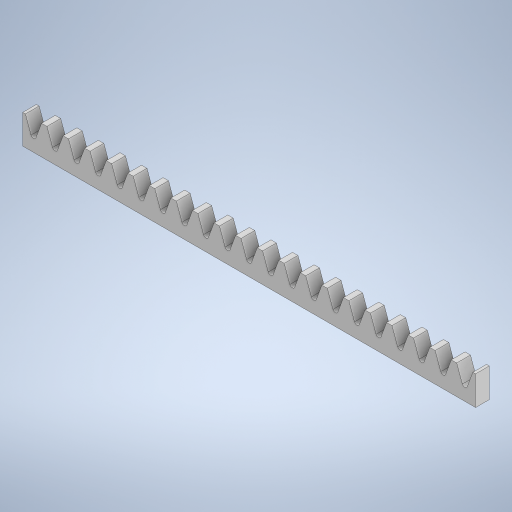
# Autodesk Inventor part: 齒條
Saved by Autodesk Inventor 2024 (Build 280153000, 153)
## iProperties
Created: 2024-04-20
Part Number: 齒條
Material: 一般
Document SubType Name: Modeling
Designer: rumse
Density: 1 g/cm^3
Appearance: 預設
Author: rumse
Autodesk Inventor part; units mm, degrees
note: some values were not read from the file. Left out: dimensions or parameters whose unit could not be read.
ref_plane "YZ Plane" through (0, 0, 0) normal (1, 0, 0) x (0, 1, 0)
ref_plane "XZ Plane" through (0, 0, 0) normal (0, 1, 0) x (-1, 0, 0)
ref_plane "XY Plane" through (0, 0, 0) normal (0, 0, 1) x (1, 0, 0)
sketch "草圖2" plane through (0, 0, 0) normal (0, 0, 1) x (1, 0, 0)
  line L0 (0, 0) -> (32.9867, 0)
  line L1 (32.9867, 0) -> (32.9867, 2.125)
  line L2 (32.9867, 2.125) -> (0, 2.125)
  line L3 (0, 2.125) -> (0, 0)
  line L4 (0, 1) -> (32.9867, 1) construction
  line L5 (0.1974, 2.125) -> (0.6069, 1)
  line L6 (0.9639, 1) -> (1.3734, 2.125)
  line L7 (0.7854, 2.125) -> (0.7854, 1) construction
  line L8 (0, 0.875) -> (32.9867, 0.875) construction
  arc A0 (0.6069, 1) -> (0.9639, 1) centre (0.7854, 1.065) ccw
  line L9 (0, 1.625) -> (32.9867, 1.625) construction
  line L10 (2.5347, 1) -> (2.9442, 2.125)
  arc A1 (2.1777, 1) -> (2.5347, 1) centre (2.3562, 1.065) ccw
  line L11 (1.7682, 2.125) -> (2.1777, 1)
  line L12 (4.1055, 1) -> (4.515, 2.125)
  arc A2 (3.7484, 1) -> (4.1055, 1) centre (3.927, 1.065) ccw
  line L13 (3.339, 2.125) -> (3.7484, 1)
  line L14 (5.6763, 1) -> (6.0858, 2.125)
  arc A3 (5.3192, 1) -> (5.6763, 1) centre (5.4978, 1.065) ccw
  line L15 (4.9098, 2.125) -> (5.3192, 1)
  line L16 (7.2471, 1) -> (7.6566, 2.125)
  arc A4 (6.89, 1) -> (7.2471, 1) centre (7.0686, 1.065) ccw
  line L17 (6.4806, 2.125) -> (6.89, 1)
  line L18 (8.8179, 1) -> (9.2274, 2.125)
  arc A5 (8.4608, 1) -> (8.8179, 1) centre (8.6394, 1.065) ccw
  line L19 (8.0514, 2.125) -> (8.4608, 1)
  line L20 (10.3887, 1) -> (10.7982, 2.125)
  arc A6 (10.0316, 1) -> (10.3887, 1) centre (10.2102, 1.065) ccw
  line L21 (9.6222, 2.125) -> (10.0316, 1)
  line L22 (11.9595, 1) -> (12.369, 2.125)
  arc A7 (11.6024, 1) -> (11.9595, 1) centre (11.781, 1.065) ccw
  line L23 (11.193, 2.125) -> (11.6024, 1)
  line L24 (13.5303, 1) -> (13.9398, 2.125)
  arc A8 (13.1732, 1) -> (13.5303, 1) centre (13.3518, 1.065) ccw
  line L25 (12.7638, 2.125) -> (13.1732, 1)
  line L26 (15.1011, 1) -> (15.5106, 2.125)
  arc A9 (14.744, 1) -> (15.1011, 1) centre (14.9226, 1.065) ccw
  line L27 (14.3346, 2.125) -> (14.744, 1)
  line L28 (16.6719, 1) -> (17.0814, 2.125)
  arc A10 (16.3148, 1) -> (16.6719, 1) centre (16.4934, 1.065) ccw
  line L29 (15.9054, 2.125) -> (16.3148, 1)
  line L30 (18.2427, 1) -> (18.6522, 2.125)
  arc A11 (17.8856, 1) -> (18.2427, 1) centre (18.0642, 1.065) ccw
  line L31 (17.4762, 2.125) -> (17.8856, 1)
  line L32 (19.8135, 1) -> (20.223, 2.125)
  arc A12 (19.4564, 1) -> (19.8135, 1) centre (19.635, 1.065) ccw
  line L33 (19.047, 2.125) -> (19.4564, 1)
  line L34 (21.3843, 1) -> (21.7938, 2.125)
  arc A13 (21.0272, 1) -> (21.3843, 1) centre (21.2058, 1.065) ccw
  line L35 (20.6177, 2.125) -> (21.0272, 1)
  line L36 (22.9551, 1) -> (23.3645, 2.125)
  arc A14 (22.598, 1) -> (22.9551, 1) centre (22.7765, 1.065) ccw
  line L37 (22.1885, 2.125) -> (22.598, 1)
  line L38 (24.5259, 1) -> (24.9353, 2.125)
  arc A15 (24.1688, 1) -> (24.5259, 1) centre (24.3473, 1.065) ccw
  line L39 (23.7593, 2.125) -> (24.1688, 1)
  line L40 (26.0967, 1) -> (26.5061, 2.125)
  arc A16 (25.7396, 1) -> (26.0967, 1) centre (25.9181, 1.065) ccw
  line L41 (25.3301, 2.125) -> (25.7396, 1)
  line L42 (27.6675, 1) -> (28.0769, 2.125)
  arc A17 (27.3104, 1) -> (27.6675, 1) centre (27.4889, 1.065) ccw
  line L43 (26.9009, 2.125) -> (27.3104, 1)
  line L44 (29.2383, 1) -> (29.6477, 2.125)
  arc A18 (28.8812, 1) -> (29.2383, 1) centre (29.0597, 1.065) ccw
  line L45 (28.4717, 2.125) -> (28.8812, 1)
  line L46 (30.8091, 1) -> (31.2185, 2.125)
  arc A19 (30.452, 1) -> (30.8091, 1) centre (30.6305, 1.065) ccw
  line L47 (30.0425, 2.125) -> (30.452, 1)
  line L48 (32.3799, 1) -> (32.7893, 2.125)
  arc A20 (32.0228, 1) -> (32.3799, 1) centre (32.2013, 1.065) ccw
  line L49 (31.6133, 2.125) -> (32.0228, 1)
  point P0 (0.7854, 0.5095)
  point P1 (0.7854, 0.875)
  point P2 (2.3562, 0.5095)
  point P3 (3.927, 0.5095)
  point P4 (5.4978, 0.5095)
  point P5 (7.0686, 0.5095)
  point P6 (8.6394, 0.5095)
  point P7 (10.2102, 0.5095)
  point P8 (11.781, 0.5095)
  point P9 (13.3518, 0.5095)
  point P10 (14.9226, 0.5095)
  point P11 (16.4934, 0.5095)
  point P12 (18.0642, 0.5095)
  point P13 (19.635, 0.5095)
  point P14 (21.2058, 0.5095)
  point P15 (22.7765, 0.5095)
  point P16 (24.3473, 0.5095)
  point P17 (25.9181, 0.5095)
  point P18 (27.4889, 0.5095)
  point P19 (29.0597, 0.5095)
  point P20 (30.6305, 0.5095)
  point P21 (32.2013, 0.5095)
  point P22 (32.7893, 2.125)
  point P23 (31.6133, 2.125)
  point P24 (31.2185, 2.125)
  point P25 (30.0425, 2.125)
  point P26 (29.6477, 2.125)
  point P27 (28.4717, 2.125)
  point P28 (28.0769, 2.125)
  point P29 (26.9009, 2.125)
  point P30 (26.5061, 2.125)
  point P31 (25.3301, 2.125)
  point P32 (24.9353, 2.125)
  point P33 (23.7593, 2.125)
  point P34 (23.3645, 2.125)
  point P35 (22.1885, 2.125)
  point P36 (21.7938, 2.125)
  point P37 (20.6177, 2.125)
  point P38 (20.223, 2.125)
  point P39 (19.047, 2.125)
  point P40 (18.6522, 2.125)
  point P41 (17.4762, 2.125)
  point P42 (17.0814, 2.125)
  point P43 (15.9054, 2.125)
  point P44 (15.5106, 2.125)
  point P45 (14.3346, 2.125)
  point P46 (13.9398, 2.125)
  point P47 (12.7638, 2.125)
  point P48 (12.369, 2.125)
  point P49 (11.193, 2.125)
  point P50 (10.7982, 2.125)
  point P51 (9.6222, 2.125)
  point P52 (9.2274, 2.125)
  point P53 (8.0514, 2.125)
  point P54 (7.6566, 2.125)
  point P55 (6.4806, 2.125)
  point P56 (6.0858, 2.125)
  point P57 (4.9098, 2.125)
  point P58 (4.515, 2.125)
  point P59 (3.339, 2.125)
  point P60 (2.9442, 2.125)
  point P61 (1.7682, 2.125)
  dimension "d17" = 32.9867
  dimension "d18" = 2.125
  dimension "d19" = 1.125
  dimension "d20" = 0.7854
  dimension "d23" = 20
  dimension "d24" = 20
  dimension "d25" = 0.125
  dimension "d26" = 0.19
  dimension "d37" = 0.5
  dimension "d40" = 1.5708
  constraints: 120 horizontal alignment, 98 end point, 51 point on line, 42 point on circle, 41 parallel, 21 centre point, 20 equal radius, 5 perpendicular, 3 tangent, 2 horizontal, 6 other
  measures "d17" distance of L1.end L3.start
  measures "d18" distance of L0.end L1.end
  measures "d20" distance of L3.start L7.start
  measures "d23" angle of L6 L7
  measures "d24" angle of L5 L7
  measures "d25" distance between parallel lines of L8 L4
  measures "d26" radius of A0
  measures "d40" distance of L6.start L10.start
extrude "擠出3" add sketch "草圖2" along normal blind 1 contours L3 L2 L5 A0 L6 L11 A1 L10 L13 A2 L12 L15 A3 L14 L17 A4 L16 L19 A5 L18 L21 A6 L20 L23 A7 L22 L25 A8 L24 L27 A9 L26 L29 A10 L28 L31 A11 L30 L33 A12 L32 L35 A13 L34 L37 A14 L36 L39 A15 L38 L41 A16 L40 L43 A17 L42 L45 A18 L44 L47 A19 L46 L49 A20 L48 L1 L0
equation "\"d17\" = rack_length"
equation "\"d19\" = whole_depth"
equation "\"d20\" = tooth_thickness"
equation "\"d23\" = pressure_angle"
equation "\"d24\" = pressure_angle"
equation "\"d25\" = rack_dedendum"
equation "\"d26\" = fillet_radius"
equation "\"d37\" = addendum"
equation "\"d40\" = circular_pitch"
equation "\"whole_depth\" = 2.25 * module"
equation "\"tooth_thickness\" = 1.5708 * module"
equation "\"circular_pitch\" = 3.14159 * module"
equation "\"addendum\" = module"
equation "\"dedendum\" = 1.25 * module"
equation "\"addendum_diameter\" = pitch_diameter + 2 * addendum"
equation "\"dedendum_diameter\" = pitch_diameter - 2 * dedendum"
equation "\"pressure_angle\" = 20deg"
equation "\"fillet_radius\" = 0.38 * module"
equation "\"rack_dedendum\" = 0.25 * module"
equation "\"rack_length\" = 32.986723"
equation "\"pitch_diameter\" = 10"
